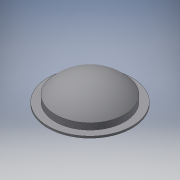
# Autodesk Inventor part: Bauteil2
Saved by Autodesk Inventor 2016 SP2 (Build 200236200, 236)
## iProperties
Created: 2018-09-27
Part Number: Bauteil2
Material: Generisch
Document SubType Name: Modeling
Designer: Nils
Density: 1 g/cm^3
Appearance: Vorgabe
Author: Nils
Autodesk Inventor part; units mm, degrees
ref_plane "YZ Plane" through (0, 0, 0) normal (1, 0, 0) x (0, 1, 0)
ref_plane "XZ Plane" through (0, 0, 0) normal (0, 1, 0) x (-1, 0, 0)
ref_plane "XY Plane" through (0, 0, 0) normal (0, 0, 1) x (1, 0, 0)
sketch "Skizze1" plane through (0, 0, 0) normal (0, 1, 0) x (-1, 0, 0)
  line L0 (27.25, -10) -> (27.25, 0) construction
  line L1 (27.25, 0) -> (-27.25, 0) construction
  line L2 (24.25, -10) -> (24.25, 0) construction
  line L3 (46, 4.8366) -> (46, 6.8366)
  line L4 (46, 6.8366) -> (38, 6.8366)
  line L5 (0, 0) -> (0, 30) construction
  line L6 (38, 6.8366) -> (38, 13.8366)
  line L7 (46, 4.8366) -> (27.75, 4.8366)
  line L8 (27.75, 4.8366) -> (27.75, 13.8366)
  line L9 (27.75, 13.8366) -> (23.75, 13.8366)
  line L10 (23.75, 13.8366) -> (23.75, 9.8366)
  line L11 (-46, 4.8366) -> (-46, 6.8366)
  line L12 (-46, 6.8366) -> (-38, 6.8366)
  line L13 (-38, 6.8366) -> (-38, 13.8366)
  line L14 (-46, 4.8366) -> (-27.75, 4.8366)
  line L15 (-27.75, 4.8366) -> (-27.75, 13.8366)
  line L16 (-27.75, 13.8366) -> (-23.75, 13.8366)
  line L17 (-23.75, 13.8366) -> (-23.75, 9.8366)
  arc A0 (38, 13.8366) -> (-38, 13.8366) centre (0, -18.6595) ccw
  line L18 (23.75, 9.8366) -> (-23.75, 9.8366)
  line L19 (0, 9.8366) -> (0, 31.3405)
  dimension "d0" = 2
  dimension "d1" = 7
  dimension "d2" = 8
  dimension "d3" = 46
  dimension "d4" = 0.5
  dimension "d5" = 0.5
  dimension "d7" = 50
  dimension "d8" = 9
  dimension "d9" = 4
  constraints: 38 end point, 8 symmetric about line, 6 vertical, 3 perpendicular, 3 point on circle, 2 horizontal, 1 centre point, 1 midpoint, 4 other
  measures "d0" distance of L3.start L3.end
  measures "d1" distance of L4.end L6.end
  measures "d2" distance of L3.end L4.end
  measures "d3" distance between parallel lines of L3 L5
  measures "d4" distance between parallel lines of L8 L0
  measures "d5" distance between parallel lines of L10 L2
  measures "d7" radius of A0
  measures "d8" distance between parallel lines of L9 L7
  measures "d9" distance between parallel lines of L9 L18
revolve "Umdrehung1" add sketch "Skizze1" angle 360 about axis through (0, 0, 9.8366) along (0, 0, 1) contours L7 L8 L9 L10 L18 L19 A0 L6 L4 L3
